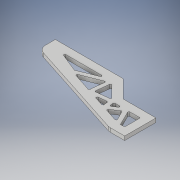
# Autodesk Inventor part: X motor supports
Saved by Autodesk Inventor 2018.2 (Build 222227000, 227)
## iProperties
Created: 2018-01-22
Part Number: X motor supports
Material: Generic
Document SubType Name: Modeling
Designer: torba
Density: 1 g/cm^3
Appearance: Default
Author: torba
Autodesk Inventor part; units mm, degrees
ref_plane "YZ Plane" through (0, 0, 0) normal (1, 0, 0) x (0, 1, 0)
ref_plane "XZ Plane" through (0, 0, 0) normal (0, 1, 0) x (-1, 0, 0)
ref_plane "XY Plane" through (0, 0, 0) normal (0, 0, 1) x (1, 0, 0)
sketch "Sketch1" plane through (0, 0, 0) normal (0, 1, 0) x (-1, 0, 0)
  line L0 (-215.9017, 85.725) -> (-215.9, 85.725)
  line L1 (-127.5447, 6.3482) -> (-156.1216, 34.925)
  line L2 (-17.7944, 6.3482) -> (-127.5447, 6.3482)
  line L3 (-127.5447, 6.3482) -> (-156.1216, 34.925) construction
  line L4 (-127.5447, 6.3482) -> (-17.7944, 6.3482) construction
  line L5 (-209.55, 34.925) -> (-156.1216, 34.925)
  line L6 (-156.1216, 34.925) -> (-127.5447, 6.3482)
  line L7 (-17.7944, 6.3482) -> (-17.7944, 85.725)
  line L8 (-17.7944, 85.725) -> (-209.55, 85.725)
  line L9 (-209.55, 34.925) -> (-209.55, 85.725)
  line L10 (-209.55, 34.925) -> (-156.1216, 34.925)
  point P0 (0, 0)
  dimension "d11" = 135
  dimension "d55" = 28.5768
  dimension "d58" = 6.3482
  dimension "d59" = 17.7945
  dimension "d60" = 85.6989
  dimension "d64" = 79.3768
  dimension "d65" = 79.3768
  dimension "d66" = 191.7555
  dimension "d67" = 198.1055
  dimension "d68" = 198.1073
  constraints: 22 end point, 4 horizontal, 3 parallel, 1 vertical
  measures "d11" angle of L4 L3
  measures "d55" distance between parallel lines of L2 L5
  measures "d58" distance from line of point (0, 0) L2
  measures "d59" distance from line of point (0, 0) L7
  measures "d60" distance from line of point (0, 0) L6
  measures "d64" distance between parallel lines of L8 L2
  measures "d65" distance between parallel lines of L2 L0
  measures "d66" distance between parallel lines of L9 L7
  measures "d67" distance from line of L0.end L7
  measures "d68" distance from line of L0.start L7
extrude "Extrusion1" add sketch "Sketch1" along normal blind 6.35
sketch "Sketch3" plane through (0, 6.35, 0) normal (0, 1, 0) x (1, 0, 0)
  line L0 (127.5447, -6.3482) -> (17.7944, -6.3482) projected
  line L1 (209.55, -34.925) -> (156.1216, -34.925) projected
  line L2 (156.1216, -34.925) -> (127.5447, -6.3482) projected
  line L3 (124.9145, -6.3482) -> (17.7944, -6.3482) projected
  line L4 (209.5517, -85.725) -> (184.1517, -85.725)
  line L5 (17.7944, -6.3482) -> (17.7944, -85.725) projected
  line L6 (17.7944, -85.725) -> (209.55, -85.725) projected
  line L7 (209.55, -85.725) -> (209.55, -34.925) projected
  line L8 (17.7944, -6.3482) -> (17.7944, -31.7482)
  line L9 (17.7944, -6.3482) -> (17.7944, -85.725) projected
  line L10 (17.7944, -31.7482) -> (184.1517, -85.725)
  line L11 (17.7944, -85.725) -> (209.55, -85.725) projected
  line L12 (184.1517, -85.725) -> (17.7944, -85.725)
  line L13 (17.7944, -85.725) -> (17.7944, -31.7482)
  point P0 (0, 0)
  point P1 (124.9145, -6.3482)
  point P2 (0, -6.35)
  dimension "d18" = 25.4
  dimension "d69" = 25.4
  dimension "d70" = 0
  dimension "d71" = 17.976
  constraints: 10 end point, 1 collinear, 1 perpendicular, 1 point on line, 1 other
  measures "d18" distance of L4.start L4.end
  measures "d69" distance of L0.end L8.end
  measures "d70" angle of L1 L4
  measures "d71" angle of L1 L10
extrude "Extrusion5" cut sketch "Sketch3" against normal through all contours L10 L6 L5
sketch "Sketch4" plane through (0, 6.35, 0) normal (0, 1, 0) x (1, 0, 0)
  line L0 (209.55, -34.925) -> (156.1216, -34.925) projected
  line L1 (156.1216, -34.925) -> (127.5447, -6.3482) projected
  line L2 (127.5447, -6.3482) -> (17.7944, -6.3482) projected
  line L3 (124.9145, -6.3482) -> (17.7944, -6.3482) projected
  line L4 (30.4944, -19.0482) -> (122.2842, -19.0482)
  line L5 (209.55, -34.925) -> (209.55, -34.925)
  line L6 (196.8504, -47.6264) -> (150.8624, -47.6264)
  line L7 (209.55, -34.925) -> (156.1216, -34.925) projected
  line L8 (209.55, -34.925) -> (209.55, -34.925)
  line L9 (196.8504, -47.6264) -> (196.8504, -73.0268)
  line L10 (150.8624, -47.6264) -> (122.2842, -19.0482)
  line L11 (184.1517, -85.725) -> (209.55, -85.725) projected
  line L12 (209.55, -85.725) -> (209.55, -34.925) projected
  line L13 (17.7944, -6.3482) -> (17.7944, -31.7482) projected
  line L14 (17.7944, -31.7482) -> (184.1517, -85.725) projected
  line L15 (17.7944, -6.3482) -> (17.7944, -31.7482) projected
  line L16 (30.4944, -19.0482) -> (30.4944, -22.5171)
  line L17 (196.8504, -73.0268) -> (186.3743, -73.0944)
  line L18 (102.9697, -46.0326) -> (30.4944, -22.5171)
  line L19 (102.9697, -46.0326) -> (186.3743, -73.0944)
  point P0 (156.1216, -34.9268)
  dimension "d89" = 0.369
  dimension "d90" = 162.024
  dimension "d91" = 12.7014
  dimension "d92" = 15.8768
  dimension "d93" = 12.6996
  dimension "d94" = 179.0556
  dimension "d95" = 12.7
  dimension "d96" = 12.7
  dimension "d99" = 0
  dimension "d100" = 0
  dimension "d101" = 11.1076
  dimension "d104" = 38.0192
  constraints: 20 end point, 5 parallel, 2 perpendicular, 2 other
  measures "d89" angle to the sketch x axis of L17
  measures "d90" angle to the sketch x axis of L18
  measures "d93" distance between parallel lines of L12 L9
  measures "d94" distance between parallel lines of L12 L16
  measures "d95" distance between parallel lines of L10 L1
  measures "d96" distance between parallel lines of L19 L14
  measures "d100" distance from line of L8.end L12
  measures "d104" distance from line of L0.start L17
extrude "Extrusion6" cut sketch "Sketch4" against normal through all contours L4 L10 L6 L9 L17 L19 L18 L16
sketch "Sketch7" plane through (0, 6.35, 0) normal (0, 1, 0) x (1, 0, 0)
  line L0 (122.2842, -19.0482) -> (30.4944, -19.0482) projected
  line L1 (30.4944, -22.5171) -> (186.3743, -73.0944) projected
  line L2 (150.8624, -47.6264) -> (122.2842, -19.0482) projected
  line L3 (122.2842, -19.0482) -> (150.8624, -47.6264) projected
  line L4 (150.8624, -47.6264) -> (196.8504, -47.6264) projected
  line L5 (196.8504, -47.6264) -> (196.8504, -73.0268) projected
  line L6 (196.8504, -73.0268) -> (186.3743, -73.0944) projected
  line L7 (186.3743, -73.0944) -> (30.4944, -22.5171) projected
  line L8 (30.4944, -22.5171) -> (30.4944, -19.0482) projected
  line L9 (30.4944, -19.0482) -> (122.2842, -19.0482) projected
  line L10 (17.7944, -31.7482) -> (184.1517, -85.725) projected
  line L11 (184.1517, -85.725) -> (209.55, -85.725) projected
  line L12 (209.55, -85.725) -> (209.55, -34.925) projected
  line L13 (209.55, -34.925) -> (156.1216, -34.925) projected
  line L14 (156.1216, -34.925) -> (127.5447, -6.3482) projected
  line L15 (127.5447, -6.3482) -> (17.7944, -6.3482) projected
  line L16 (17.7944, -6.3482) -> (17.7944, -31.7482) projected
  line L17 (122.2842, -19.0482) -> (118.7272, -51.1454)
  line L18 (122.2842, -19.0482) -> (76.3893, -37.4083)
  line L19 (76.3893, -37.4083) -> (30.4944, -19.0482)
  line L20 (150.8624, -47.6264) -> (118.7272, -51.1454)
  line L21 (150.8624, -47.6264) -> (196.8504, -47.6264) projected
  line L22 (173.8564, -47.6264) -> (186.3743, -73.0944)
  line L23 (152.4496, -62.1205) -> (173.8564, -47.6264)
  line L24 (152.4496, -62.1205) -> (150.8624, -47.6264)
  line L25 (186.3743, -73.0944) -> (196.8504, -73.0268) projected
  line L26 (186.3743, -73.0944) -> (173.8564, -47.6264) construction
  line L27 (189.2238, -71.6938) -> (176.7058, -46.2258)
  line L28 (171.007, -49.0269) -> (183.5249, -74.4949)
  arc A0 (183.5249, -74.4949) -> (189.2238, -71.6938) centre (186.3743, -73.0944) ccw
  arc A1 (176.7058, -46.2258) -> (171.007, -49.0269) centre (173.8564, -47.6264) ccw
  line L29 (173.8564, -47.6264) -> (152.4496, -62.1205) construction
  line L30 (172.0763, -44.9973) -> (150.6695, -59.4915)
  line L31 (154.2297, -64.7496) -> (175.6365, -50.2554)
  arc A2 (175.6365, -50.2554) -> (172.0763, -44.9973) centre (173.8564, -47.6264) ccw
  arc A3 (150.6695, -59.4915) -> (154.2297, -64.7496) centre (152.4496, -62.1205) ccw
  line L32 (152.4496, -62.1205) -> (150.8624, -47.6264) construction
  line L33 (155.6058, -61.7749) -> (154.0186, -47.2807)
  line L34 (147.7063, -47.972) -> (149.2935, -62.4661)
  arc A4 (149.2935, -62.4661) -> (155.6058, -61.7749) centre (152.4496, -62.1205) ccw
  arc A5 (154.0186, -47.2807) -> (147.7063, -47.972) centre (150.8624, -47.6264) ccw
  line L35 (150.8624, -47.6264) -> (118.7272, -51.1454) construction
  line L36 (150.5168, -44.4702) -> (118.3816, -47.9892)
  line L37 (119.0729, -54.3015) -> (151.208, -50.7825)
  arc A6 (151.208, -50.7825) -> (150.5168, -44.4702) centre (150.8624, -47.6264) ccw
  arc A7 (118.3816, -47.9892) -> (119.0729, -54.3015) centre (118.7272, -51.1454) ccw
  line L38 (118.7272, -51.1454) -> (122.2842, -19.0482) construction
  line L39 (121.8829, -51.4951) -> (125.4399, -19.3979)
  line L40 (119.1285, -18.6985) -> (115.5716, -50.7957)
  arc A8 (115.5716, -50.7957) -> (121.8829, -51.4951) centre (118.7272, -51.1454) ccw
  arc A9 (125.4399, -19.3979) -> (119.1285, -18.6985) centre (122.2842, -19.0482) ccw
  line L41 (122.2842, -19.0482) -> (76.3893, -37.4083) construction
  line L42 (121.1049, -16.1003) -> (75.2101, -34.4604)
  line L43 (77.5686, -40.3561) -> (123.4635, -21.996)
  arc A10 (123.4635, -21.996) -> (121.1049, -16.1003) centre (122.2842, -19.0482) ccw
  arc A11 (75.2101, -34.4604) -> (77.5686, -40.3561) centre (76.3893, -37.4083) ccw
  line L44 (76.3893, -37.4083) -> (30.4944, -19.0482) construction
  line L45 (77.5686, -34.4604) -> (31.6737, -16.1003)
  line L46 (29.3152, -21.996) -> (75.2101, -40.3561)
  arc A12 (75.2101, -40.3561) -> (77.5686, -34.4604) centre (76.3893, -37.4083) ccw
  arc A13 (31.6737, -16.1003) -> (29.3152, -21.996) centre (30.4944, -19.0482) ccw
  point P0 (0, 0)
  point P1 (180.1154, -60.3604)
  point P2 (163.153, -54.8734)
  point P3 (151.656, -54.8734)
  point P4 (134.7948, -49.3859)
  point P5 (120.5057, -35.0968)
  point P6 (99.3368, -28.2282)
  point P7 (53.4419, -28.2282)
  dimension "d109" = 6.35
  dimension "d110" = 6.35
  dimension "d111" = 6.35
  dimension "d112" = 6.35
  dimension "d113" = 6.35
  dimension "d114" = 6.35
  dimension "d115" = 6.35
  constraints: 70 end point, 28 point on circle, 28 tangent, 14 centre point, 9 equal length, 8 midpoint, 4 point on line, 1 perpendicular
  measures "d109" diameter of A1
  measures "d110" diameter of A3
  measures "d111" diameter of A5
  measures "d112" diameter of A7
  measures "d113" diameter of A9
  measures "d114" diameter of A11
  measures "d115" diameter of A13
extrude "Extrusion7" add sketch "Sketch7" against normal blind 6.35 contours L18 L40 L0 | L0 L40 A9 A10 L2 | L2 A10 L43 L17 | L17 L43 L40 L18 | L40 L18 A12 L45 L42 L0 | L0 L42 A9 L40 | A10 L39 L2 | L2 L39 L36 L17 L43 A10 | L17 L36 A7 L1 L40 L43 | L40 L43 L1 A12 L18 | L36 L39 L20 L17 | L17 L1 A7 L36 | A12 L1 L18 | L18 L19 A11 L42 L45 A12 | L45 L42 A11 L19 L0 | L0 L8 L46 A13 L45 | L36 A5 L2 | L2 A5 L20 L39 L36 | L1 A8 A7 | L20 L39 A8 L1 | L1 A7 L40 | L43 A12 L1 | L1 A12 A11 | L1 A11 L19 | L19 A11 L1 L46 L8 | A5 A6 L4 L2 | L2 L20 A5 | L20 L34 L37 L1 A8 L39 | L1 L37 A8 | A11 L46 L1 | L24 L37 L34 L20 | L4 A6 L24 | L33 L4 A6 | L4 L33 L30 L24 A6 | L24 L30 A3 L1 L34 L37 | L1 A3 L34 | L30 L33 L23 L1 L24 | L24 L1 A3 L30 | L30 A1 L4 | L4 A1 L28 L23 L33 L30 | L1 L24 L23 A4 A3 | L1 L23 L24 | A1 A2 L4 | L4 L23 L28 A1 | L33 A4 L1 L23 | L23 L28 L31 L1 A4 L33 | A4 L1 L31 | L4 A2 L31 L22 | L22 L31 L28 L23 | L27 L4 A2 | L4 L27 A0 L6 L22 L31 A2 | L22 L1 L28 L31 | L1 L6 A0 L28
fillet "Fillet5" radius 1.5875 22 edges at (196.8504, 3.175, 47.6264) (196.8504, 3.175, 73.0268) (182.1653, 3.175, 71.7287) (189.5493, 3.175, 73.0739) (177.3942, 3.175, 47.6264) (172.6161, 3.175, 52.3005) (168.1934, 3.175, 47.6264) (154.0564, 3.175, 47.6264) (122.3192, 3.175, 47.558) (81.1093, 3.175, 38.9397) (76.3893, 3.175, 33.9886) (115.6437, 3.175, 50.1449) (126.0872, 3.175, 53.5334) (125.16, 3.175, 21.9239) (147.9837, 3.175, 44.7476) (113.7361, 3.175, 19.0482) (39.0425, 3.175, 19.0482) (149.1342, 3.175, 61.0113) (156.3115, 3.175, 63.3401) (155.0322, 3.175, 56.5376) (148.0519, 3.175, 51.1281) (118.5451, 3.175, 23.9636)
fillet "Fillet6" radius 12.7 2 edges at (184.1517, 3.175, 85.725) (17.7944, 3.175, 31.7482)
sketch "Sketch8" plane through (0, 6.35, 0) normal (0, 1, 0) x (1, 0, 0)
  circle A0 centre (32.6885, -24.3071) radius 4.605
  point P0 (0, 0)
  dimension "d120" = 9.2099
  dimension "d121" = 40.7355
  constraints: 1 centre point
  measures "d120" diameter of A0
  measures "d121" distance of A0.centre point (0, 0)
extrude "Extrusion8" add sketch "Sketch8" against normal blind 6.35
body "Solid1"
